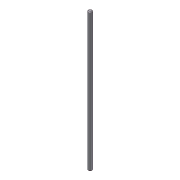
# Autodesk Inventor part: FOX-ME-123
Saved by Autodesk Inventor 2014 SP1 (Build 180222100, 222)
## iProperties
Created: 2012-08-03
Part Number: FOX-ME-123
Document SubType Name: Modeling
Designer: Robert Davis
Density: 8.08 g/cm^3
Material: Stainless Steel
Mass: 4.96575 g
Surface Area: 8.73735 cm^2
Volume: 0.614573 cm^3
Description: THREADED ROD
Appearance: Steel
Author: Robert Davis
Autodesk Inventor part; units mm, degrees
ref_plane "YZ Plane" through (0, 0, 0) normal (1, 0, 0) x (0, 1, 0)
ref_plane "XZ Plane" through (0, 0, 0) normal (0, 1, 0) x (-1, 0, 0)
ref_plane "XY Plane" through (0, 0, 0) normal (0, 0, 1) x (1, 0, 0)
sketch "Sketch1" plane through (0, 0, 0) normal (0, 0, 1) x (1, 0, 0)
  circle A0 centre (0, 0) radius 1.4224
  dimension "d0" = 2.8448
  constraints: 1 centre point
  measures "d0" diameter of A0
extrude "Extrusion1" add sketch "Sketch1" along normal mid plane 98
chamfer "Chamfer1" distance 0.5 angle 45 2 edges at (-1.4224, 0, 49) (-1.4224, 0, -49)
body "Solid1"
